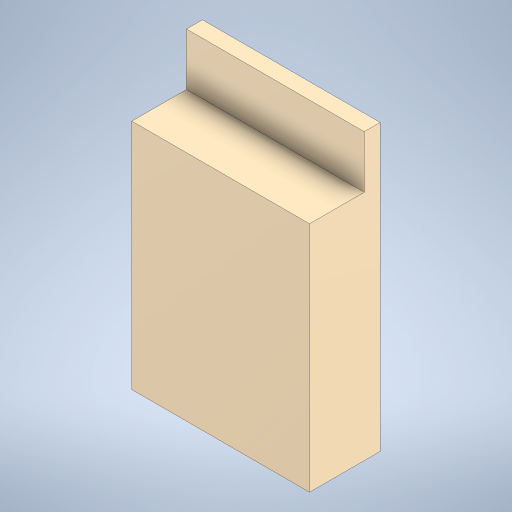
# Autodesk Inventor part: DHT22
Saved by Autodesk Inventor 2023 (Build 270158000, 158)
## iProperties
Created: 2023-09-21
Part Number: DHT22
Material: Generic
Document SubType Name: Modeling
Designer: Gage
Density: 1 g/cm^3
Appearance: Default
Author: Gage
Autodesk Inventor part; units mm, degrees
ref_plane "YZ Plane" through (0, 0, 0) normal (1, 0, 0) x (0, 1, 0)
ref_plane "XZ Plane" through (0, 0, 0) normal (0, 1, 0) x (-1, 0, 0)
ref_plane "XY Plane" through (0, 0, 0) normal (0, 0, 1) x (1, 0, 0)
sketch "Sketch1" plane through (0, 0, 0) normal (0, 1, 0) x (-1, 0, 0)
  line L0 (7.7391, -3.0758) -> (-7.7391, -3.0758)
  line L1 (-7.7391, -3.0758) -> (-7.7391, 3.0758)
  line L2 (-7.7391, 3.0758) -> (7.7391, 3.0758)
  line L3 (7.7391, 3.0758) -> (7.7391, -3.0758)
  point P0 (0, 0)
  point P1 (-7.7391, 0)
  point P2 (0, -3.0758)
  dimension "d0" = 15.4781
  dimension "d1" = 6.1516
  constraints: 8 end point, 2 midpoint, 2 parallel, 1 horizontal, 1 horizontal alignment, 1 perpendicular, 1 vertical alignment
  measures "d0" distance of L1.end L2.end
  measures "d1" distance of L0.end L1.end
extrude "Extrusion1" add sketch "Sketch1" along normal blind 20.2406
sketch "Sketch2" plane through (0, 20.2406, 0) normal (0, 1, 0) x (1, 0, 0)
  line L0 (-7.7391, 3.0758) -> (-7.7391, -3.0758) projected
  line L1 (7.7391, -3.0758) -> (7.7391, 3.0758) projected
  line L2 (-7.7391, 3.0758) -> (7.7391, 3.0758)
  line L3 (7.7391, 3.0758) -> (7.7391, 1.6867)
  line L4 (7.7391, 1.6867) -> (-7.7391, 1.6867)
  line L5 (-7.7391, 1.6867) -> (-7.7391, 3.0758)
  point P0 (0, 0)
  point P1 (-7.7391, 1.6867)
  dimension "d4" = 1.3891
  constraints: 8 end point, 2 parallel, 1 horizontal, 1 perpendicular, 1 point on line
  measures "d4" distance between parallel lines of L4 L2
extrude "Extrusion2" add sketch "Sketch2" along normal blind 4.5641
sketch "Sketch3" plane through (-7.7391, 20.2406, -1.6867) normal (0, 0, 1) x (1, 0, 0)
  point P0 (7.7391, -20.2406)
body "Solid1"
